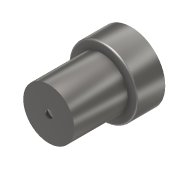
# Autodesk Inventor part: Musab4
Saved by Autodesk Inventor 2017 (Build 210142000, 142)
## iProperties
Created: 2017-09-15
Part Number: Musab4
Material: Steel, Alloy
Document SubType Name: Modeling
Designer: Amer Mohia
Density: 7.73 g/cm^3
Appearance: Semi-Polished
Author: Amer Mohia
Autodesk Inventor part; units mm, degrees
ref_plane "YZ Plane" through (0, 0, 0) normal (1, 0, 0) x (0, 1, 0)
ref_plane "XZ Plane" through (0, 0, 0) normal (0, 1, 0) x (-1, 0, 0)
ref_plane "XY Plane" through (0, 0, 0) normal (0, 0, 1) x (1, 0, 0)
sketch "Sketch1" plane through (0, 0, 0) normal (0, 0, 1) x (1, 0, 0)
  line L0 (-1.2723, 5.8241) -> (-1.2723, -4.8856)
  line L1 (1.2277, 5.0871) -> (1.2277, 3.0871)
  line L2 (5.7277, 5.0871) -> (5.7277, -0.9129)
  line L3 (3.9777, -0.9129) -> (3.9777, -11.9129)
  line L4 (1.2277, 5.0871) -> (5.7277, 5.0871)
  line L5 (5.7277, -0.9129) -> (3.9777, -0.9129)
  line L6 (0.7277, 3.0871) -> (0.7277, -7.8065)
  line L7 (1.2277, 3.0871) -> (0.7277, 3.0871)
  line L8 (0.7277, -7.8065) -> (2.9777, -7.8065)
  line L9 (2.9777, -7.8065) -> (2.9777, -10.8065)
  line L10 (0.0277, -11.0469) -> (-0.4723, -11.9129)
  line L11 (-0.4723, -11.9129) -> (3.9777, -11.9129)
  line L12 (2.9777, -10.8065) -> (0.1665, -10.8065)
  line L13 (0.1665, -10.8065) -> (0.0277, -11.0469)
  point P0 (0, 0)
  dimension "d0" = 5
  dimension "d1" = 6
  dimension "d2" = 14
  dimension "d3" = 11
  dimension "d4" = 2
  dimension "d5" = 4
  dimension "d6" = 10.5
  dimension "d7" = 3
  dimension "d8" = 8.5
  dimension "d11" = 0.8
  constraints: 28 end point, 5 horizontal, 5 vertical, 2 horizontal alignment, 1 parallel, 1 perpendicular
  measures "d0" diameter of L1 L0
  measures "d1" distance of L2.start L2.end
  measures "d2" diameter of L2 L0
  measures "d3" distance of L3.start L3.end
  measures "d4" distance of L1.start L1.end
  measures "d5" diameter of L6 L0
  measures "d6" diameter of L3 L0
  measures "d7" distance of L8.end L9.end
  measures "d8" diameter of L9 L0
  measures "d11" horizontal distance of L0.end L10.end
revolve "Revolution1" add sketch "Sketch1" angle 360 about axis through (-1.2723, 5.8241, 0) along (0, -1, 0)
fillet "Fillet1" radius 0.5 1 edges at (-8.2723, -0.9129, 0)
sketch "Sketch4" plane through (-1.2723, 5.0871, 0) normal (0, 1, 0) x (1, 0, 0)
  circle A0 centre (-4.85, 0) radius 0.65
  circle A1 centre (4.85, 0) radius 0.65
  circle A2 centre (0, 0) radius 7 projected
  point P0 (1.2723, 0)
  dimension "d25" = 1.3
  dimension "d26" = 1.3
  dimension "d28" = 1.5
  dimension "d29" = 1.5
  dimension "d30" = 11
  constraints: 2 centre point
  measures "d25" diameter of A0
  measures "d26" diameter of A1
sketch "Sketch5" plane through (0, 0, 0) normal (0, 0, 1) x (1, 0, 0)
  line L0 (-8.2723, 5.0871) -> (5.7277, 5.0871) projected
  line L1 (3.5777, 5.0871) -> (1.9777, -8.3912)
  line L2 (-8.2723, 5.0871) -> (-8.2723, -0.4129) projected
  line L3 (5.7277, 5.0871) -> (5.7277, -0.4129) projected
  line L4 (-6.1223, 5.0871) -> (-4.5223, -8.3912)
  line L5 (-5.5223, -10.8065) -> (-5.5223, -7.8065) projected
  line L6 (2.9777, -10.8065) -> (2.9777, -7.8065) projected
  point P0 (0, 0)
  dimension "d31" = 2.15
  dimension "d32" = 2.15
  dimension "d33" = 1
  dimension "d34" = 1
  constraints: 4 end point, 2 point on line
  measures "d31" distance from line of L3 L1.start
  measures "d32" distance from line of L2 L4.start
  measures "d33" distance from line of L6 L1.end
  measures "d34" distance from line of L5 L4.end
sweep "Sweep2" cut profiles "Sketch4" path "Sketch5" path curves L1 contours A1
sketch "Sketch6" plane through (-1.2723, 5.0871, 0) normal (0, 1, 0) x (1, 0, 0)
  circle A0 centre (-4.85, 0) radius 0.65
  circle A1 centre (0, 0) radius 7 projected
  circle A2 centre (4.85, 0) radius 0.65 projected
  point P0 (1.2723, 0)
  dimension "d37" = 1.3
  dimension "d38" = 11
  constraints: 1 centre point
  measures "d37" diameter of A0
sketch "Sketch7" plane through (0, 0, 0) normal (0, 0, 1) x (1, 0, 0)
  line L0 (-8.2723, 5.0871) -> (5.7277, 5.0871) projected
  line L1 (-6.1223, 5.0871) -> (-4.5223, -8.1262)
  line L2 (-5.5223, -10.8065) -> (2.9777, -10.8065) projected
  line L3 (-5.5223, -7.8065) -> (2.9777, -7.8065) projected
  line L4 (-5.5223, -10.8065) -> (-5.5223, -7.8065) projected
  line L5 (-8.2723, 5.0871) -> (-8.2723, -0.4129) projected
  point P0 (0, 0)
  dimension "d39" = 1
  dimension "d40" = 2.15
  constraints: 2 end point, 1 point on line
  measures "d39" distance from line of L4 L1.end
  measures "d40" distance from line of L5 L1.start
sweep "Sweep3" cut profiles "Sketch6" path "Sketch7" path curves L1 contours A0
body "Solid1"
